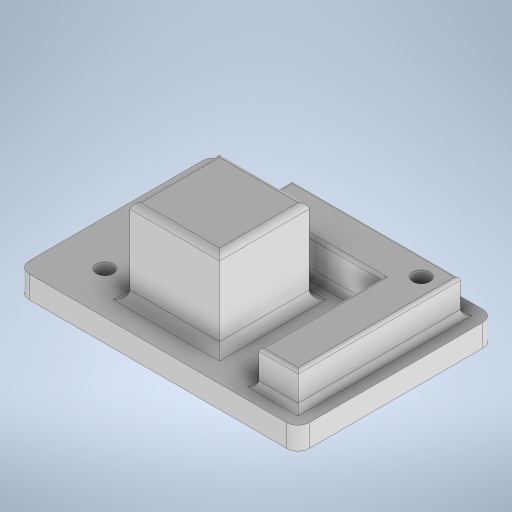
# Autodesk Inventor part: Screwing_plate
Saved by Autodesk Inventor 2024.3 (Build 283343000, 343)
## iProperties
Created: 2025-07-30
Part Number: Screwing_plate
Material: Generico
Document SubType Name: Modeling
Designer: chris
Density: 1 g/cm^3
Appearance: Default
Author: chris
Autodesk Inventor part; units mm, degrees
ref_plane "YZ Plane" through (0, 0, 0) normal (1, 0, 0) x (0, 1, 0)
ref_plane "XZ Plane" through (0, 0, 0) normal (0, 1, 0) x (-1, 0, 0)
ref_plane "XY Plane" through (0, 0, 0) normal (0, 0, 1) x (1, 0, 0)
sketch "Schizzo1" plane through (0, 0, 0) normal (0, 0, 1) x (1, 0, 0)
  line L0 (0.175, 0.25) -> (-0.175, 0.25)
  line L1 (-0.175, 0.25) -> (-0.175, -0.25)
  line L2 (-0.175, -0.25) -> (0.175, -0.25)
  line L3 (0.175, -0.25) -> (0.175, 0.25)
  line L4 (0.175, 0.25) -> (-0.175, -0.25) construction
  line L5 (-0.175, 0.25) -> (0.175, -0.25) construction
  point P0 (0, 0)
  dimension "d0" = 0.5
  dimension "d1" = 0.35
  constraints: 12 end point, 2 midpoint, 2 parallel, 1 horizontal, 1 perpendicular
  measures "d0" distance of L0.end L1.end
  measures "d1" distance of L1.end L2.end
extrude "Estrusione1" add sketch "Schizzo1" along normal blind 0.04
sketch "Schizzo2" plane through (0, 0, 0.04) normal (0, 0, 1) x (1, 0, 0)
  line L0 (-0.175, 0.25) -> (-0.175, -0.25) construction
  line L1 (-0.175, -0.25) -> (0.175, -0.25) construction
  line L2 (0.175, -0.25) -> (0.175, 0.25) construction
  line L3 (0.175, 0.25) -> (-0.175, 0.25) construction
  line L4 (-0.145, -0.08) -> (-0.075, -0.08)
  line L5 (-0.075, -0.08) -> (-0.075, 0.22)
  line L6 (-0.075, 0.22) -> (-0.145, 0.22)
  line L7 (-0.145, 0.22) -> (-0.145, -0.08)
  point P0 (0, 0)
  dimension "d4" = 0.03
  dimension "d5" = 0.03
  dimension "d6" = 0.07
  dimension "d7" = 0.3
  constraints: 8 end point, 2 parallel, 1 horizontal, 1 perpendicular
  measures "d4" distance between parallel lines of L0 L7
  measures "d5" distance between parallel lines of L3 L6
  measures "d6" distance of L4.start L4.end
  measures "d7" distance of L6.end L4.start
extrude "Estrusione2" add sketch "Schizzo2" along normal blind 0.06
sketch "Schizzo3" plane through (0, 0, 0.04) normal (0, 0, 1) x (1, 0, 0)
  line L0 (-0.075, -0.08) -> (-0.145, -0.08) construction
  line L1 (-0.145, -0.08) -> (-0.145, 0.22) construction
  line L2 (-0.145, 0.22) -> (-0.075, 0.22) construction
  line L3 (-0.075, 0.22) -> (-0.075, -0.08) construction
  line L4 (-0.175, 0.25) -> (-0.175, -0.25) construction
  line L5 (-0.175, -0.25) -> (0.175, -0.25) construction
  line L6 (0.175, -0.25) -> (0.175, 0.25) construction
  line L7 (0.175, 0.25) -> (-0.175, 0.25) construction
  line L8 (-0.075, 0.15) -> (0.145, 0.15)
  line L9 (0.145, 0.15) -> (0.145, 0.22)
  line L10 (0.145, 0.22) -> (-0.075, 0.22)
  line L11 (-0.075, 0.22) -> (-0.075, 0.15)
  line L12 (-0.075, -0.08) -> (-0.075, 0.22) projected
  line L13 (-0.075, 0.22) -> (-0.145, 0.22) projected
  point P0 (0, 0)
  dimension "d10" = 0.03
  dimension "d11" = 0.07
  constraints: 8 end point, 2 collinear, 2 parallel, 1 horizontal, 1 perpendicular
  measures "d10" distance between parallel lines of L6 L9
  measures "d11" distance of L8.end L9.end
extrude "Estrusione3" add sketch "Schizzo3" along normal blind 0.06
sketch "Schizzo4" plane through (0, 0, 0.04) normal (0, 0, 1) x (1, 0, 0)
  line L0 (-0.035, -0.1) -> (0.125, -0.1)
  line L1 (0.125, -0.1) -> (0.125, 0.06)
  line L2 (0.125, 0.06) -> (-0.035, 0.06)
  line L3 (-0.035, 0.06) -> (-0.035, -0.1)
  line L4 (-0.175, 0.25) -> (-0.175, -0.25) construction
  line L5 (-0.175, -0.25) -> (0.175, -0.25) construction
  line L6 (0.175, -0.25) -> (0.175, 0.25) construction
  line L7 (0.175, 0.25) -> (-0.175, 0.25) construction
  line L8 (-0.145, 0.22) -> (0.145, 0.22) construction
  line L9 (0.145, 0.22) -> (0.145, 0.15) construction
  line L10 (0.145, 0.15) -> (-0.075, 0.15) construction
  line L11 (-0.075, 0.15) -> (-0.075, -0.08) construction
  line L12 (-0.075, -0.08) -> (-0.145, -0.08) construction
  line L13 (-0.145, -0.08) -> (-0.145, 0.22) construction
  point P0 (0, 0)
  dimension "d14" = 0.16
  dimension "d15" = 0.16
  dimension "d16" = 0.05
  dimension "d17" = 0.15
  constraints: 8 end point, 2 parallel, 1 horizontal, 1 perpendicular
  measures "d14" distance of L0.end L1.end
  measures "d15" distance of L0.start L0.end
  measures "d16" distance between parallel lines of L6 L1
  measures "d17" distance between parallel lines of L5 L0
extrude "Estrusione4" add sketch "Schizzo4" along normal blind 0.15
sketch "Schizzo5" plane through (0, 0, 0.04) normal (0, 0, 1) x (1, 0, 0)
  line L0 (0.125, -0.1) -> (-0.035, -0.1) construction
  line L1 (-0.035, -0.1) -> (-0.035, 0.06) construction
  line L2 (-0.035, 0.06) -> (0.125, 0.06) construction
  line L3 (0.125, 0.06) -> (0.125, -0.1) construction
  line L4 (-0.175, 0.25) -> (-0.175, -0.25) construction
  line L5 (-0.175, -0.25) -> (0.175, -0.25) construction
  line L6 (0.175, -0.25) -> (0.175, 0.25) construction
  line L7 (0.175, 0.25) -> (-0.175, 0.25) construction
  line L8 (-0.145, 0.22) -> (0.145, 0.22) construction
  line L9 (0.145, 0.22) -> (0.145, 0.15) construction
  line L10 (0.145, 0.15) -> (-0.075, 0.15) construction
  line L11 (-0.075, 0.15) -> (-0.075, -0.08) construction
  line L12 (-0.075, -0.08) -> (-0.145, -0.08) construction
  line L13 (-0.145, -0.08) -> (-0.145, 0.22) construction
  line L14 (0.125, -0.1) -> (0.125, 0.06) construction
  line L15 (0.125, 0.06) -> (-0.035, 0.06) construction
  line L16 (-0.035, 0.06) -> (-0.035, -0.1) construction
  line L17 (-0.035, -0.1) -> (0.125, -0.1) construction
  line L18 (-0.075, -0.08) -> (-0.075, 0.15) construction
  line L19 (-0.075, 0.15) -> (0.145, 0.15) construction
  line L20 (0.145, 0.15) -> (0.145, 0.22) construction
  line L21 (0.145, 0.22) -> (-0.145, 0.22) construction
  line L22 (-0.145, 0.22) -> (-0.145, -0.08) construction
  line L23 (-0.145, -0.08) -> (-0.075, -0.08) construction
  line L24 (-0.145, -0.08) -> (-0.075, -0.08) projected
  point P0 (0, 0)
  point P1 (-0.1, -0.17)
  point P2 (0.1, -0.17)
  point P3 (-0.11, -0.08)
  dimension "d20" = 0.08
  dimension "d21" = 0.2
  dimension "d22" = 0.075
  constraints: 1 horizontal alignment, 1 midpoint
  measures "d20" distance from line of L5 point (-0.1, -0.17)
  measures "d21" distance of point (0.1, -0.17) point (-0.1, -0.17)
  measures "d22" distance from line of L4 point (-0.1, -0.17)
hole "Foro1" at (-0.1, -0.17, 0.04) at (0.1, -0.17, 0.04) direction (0, 0, -1) diameter 0.03 depth 0.02 tip angle 118
sketch "Schizzo6" plane through (0, 0, 0.1) normal (0, 0, 1) x (1, 0, 0)
  line L0 (-0.075, -0.08) -> (-0.075, 0.15) construction
  line L1 (-0.075, 0.15) -> (0.145, 0.15) construction
  line L2 (0.145, 0.15) -> (0.145, 0.22) construction
  line L3 (0.145, 0.22) -> (-0.145, 0.22) construction
  line L4 (-0.145, 0.22) -> (-0.145, -0.08) construction
  line L5 (-0.145, -0.08) -> (-0.075, -0.08) construction
  point P0 (0, 0)
  point P1 (-0.11, 0.185)
  point P2 (0.145, 0.185)
  point P3 (-0.11, -0.08)
  constraints: 2 midpoint, 1 horizontal alignment, 1 vertical alignment
hole "Foro2" at (-0.11, 0.185, 0.1) direction (0, 0, -1) diameter 0.03 depth 0.02 tip angle 118
fillet "Raccordo1" radius 0.02 4 edges at (0.175, 0.25, 0.02) (-0.175, 0.25, 0.02) (0.175, -0.25, 0.02) (-0.175, -0.25, 0.02)
fillet "Raccordo2" radius 0.015 4 edges at (0.125, -0.02, 0.04) (0.045, -0.1, 0.04) (-0.035, -0.02, 0.04) (0.045, 0.06, 0.04)
fillet "Raccordo3" radius 0.01 4 edges at (0.045, -0.1, 0.19) (-0.035, -0.02, 0.19) (0.045, 0.06, 0.19) (0.125, -0.02, 0.19)
fillet "Raccordo4" radius 0.01 6 edges at (-0.075, 0.035, 0.04) (0.035, 0.15, 0.04) (0.145, 0.185, 0.04) (0, 0.22, 0.04) (-0.145, 0.07, 0.04) (-0.11, -0.08, 0.04)
fillet "Raccordo5" radius 0.005 6 edges at (-0.075, 0.035, 0.1) (0.035, 0.15, 0.1) (0.145, 0.185, 0.1) (0, 0.22, 0.1) (-0.145, 0.07, 0.1) (-0.11, -0.08, 0.1)
